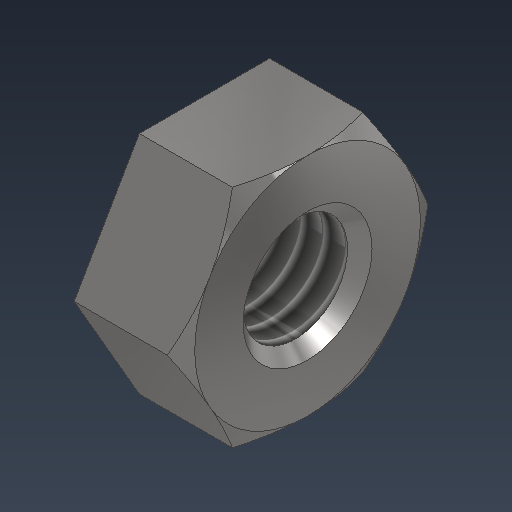
# Autodesk Inventor part: LBNR4
Saved by Autodesk Inventor 2021 (Build 250183000, 183)
## iProperties
Part Number: LBNR4
Material: 鋼、炭素鋼
Catalog Web Link: www.cadenas.de
Description: LBNR, LBNL, SLBNR, SLBNL, KNTR, KNTL, SKNTR-Nuts
Vendor: MISUMI
Document SubType Name: Modeling
Designer: partserver
Manufacturer: MISUMI
Mass: 0.843306 g
Surface Area: 1.72411 cm^2
Volume: 0.107428 cm^3
Density: 7.85 g/cm^3
Appearance: 半つや出し
Category: PARTsolutions
Company: MISUMI
PSOL_IDENT_0: {$CADENAS_DATA\23d-libs\misumi\metric\27_screws_nuts\slbnl.prj},197 {VTYP=3D},{NB=LBNR4},{LINA=LBNR4
PSOL_IDENT_1: },{NN=LBNR, LBNL, SLBNR, SLBNL, KNTR, KNTL, SKNTR},{DATE=09.09.2019 15:27:56},{GEOMDATE=05.11.2010 0
PSOL_IDENT_2: 0:00:00},{VERSION=},{LINEID=30},{WBVAR=TRS,MAT,CS},{WBNUMERIC=}  {NB=LBNR4},{LINA=LBNR4},{KT=DUMMY},
PSOL_IDENT_3: {PN=LBNR4},{TS=LBN},{TRS=R},{MAT=},{ST=Trivalent Chromate},{CS=1},{M1=4},{M=4.0},{P=0.70},{B=7.0},{E
PSOL_IDENT_4: E=8.1},{T=3.2},{T1=0.0},{TFX=3.2},{T1FX=2.4},{CALG='1','JIS Class 1','2','JIS Class 3'},{TRSALG= 'R'
PSOL_IDENT_5: , 'Right-Hand Thread', 'L', 'Left-Hand Thread' },{MATALG= '', 'SWCH Carbon Steel', 'S', '304 Stainle
PSOL_IDENT_6: ss Steel' }
NB: LBNR4
NN: LBNR, LBNL, SLBNR, SLBNL, KNTR, KNTL, SKNTR
NT: Nuts
NBSYN: $PN.
LINA: LBNR4
CATALOG: Misumi
PN: LBNR4
TRS: Right-Hand Thread
MAT: JIS-SWCH Carbon Steel Equivalent
ST: Trivalent Chromate
CS: JIS Class 1
M1: 4
P: 0.7
B: 7
EE: 8.1
T: 3.2
T1: 0
SUPPLIER: MISUMI
ARTICLENO: LBNR4
BOMINFO: LBNR4
CREATOR: CADENAS GmbH
Title: LBNR4
Author: Cadenas PARTsolutions
Comments: Nuts
Autodesk Inventor part; units mm, degrees
sketch "Sketch_1" plane through (0, 0, 0) normal (0, 0, 1) x (1, 0, 0)
  line L0 (1.6, 0) -> (-1.6, 0)
  line L1 (-1.6, 0) -> (-1.6, 3.5)
  line L2 (-1.6, 3.5) -> (-1.2825, 4.05)
  line L3 (-1.2825, 4.05) -> (1.6, 4.05)
  line L4 (1.6, 4.05) -> (1.6, 0)
  line L5 (1.6, 0) -> (-1.6, 0)
  constraints: 12 end point
revolve "Revolution1" add sketch "Sketch_1" angle 360 about axis through (1.6, 0, 0) along (1, 0, 0)
sketch "Sketch_2" plane through (0, 0, 0) normal (0, 0, 1) x (1, 0, 0)
  line L0 (1.6, 0) -> (-1.6, 0)
  line L1 (-1.6, 0) -> (-1.6, 2)
  line L2 (-1.6, 2) -> (-1.221, 1.621)
  line L3 (-1.221, 1.621) -> (1.221, 1.621)
  line L4 (1.221, 1.621) -> (1.6, 2)
  line L5 (1.6, 2) -> (1.6, 0)
  line L6 (1.6, 0) -> (-1.6, 0)
  constraints: 14 end point
revolve "Revolution2" cut sketch "Sketch_2" angle 360 about axis through (1.6, 0, 0) along (1, 0, 0)
thread "Thread1" size "M4x0.7" class "6H" standard "ISO Metric profile" full length
sketch "Sketch_3" plane through (0, 0, 0) normal (1, 0, 0) x (0, 1, 0)
  line L0 (-7, 7) -> (-7, -7)
  line L1 (-7, -7) -> (7, -7)
  line L2 (7, -7) -> (7, 7)
  line L3 (7, 7) -> (-7, 7)
  line L4 (-2.0207, 3.5) -> (-4.0415, 0)
  line L5 (-4.0415, 0) -> (-2.0207, -3.5)
  line L6 (-2.0207, -3.5) -> (2.0207, -3.5)
  line L7 (2.0207, -3.5) -> (4.0415, 0)
  line L8 (4.0415, 0) -> (2.0207, 3.5)
  line L9 (2.0207, 3.5) -> (-2.0207, 3.5)
  constraints: 20 end point
extrude "Extrusion1" cut sketch "Sketch_3" along normal mid plane 3.2
ref_plane "cp_XY" through (1.6, 0, 0) normal (1, 0, 0) x (0, 0, -1)
ref_plane "cp_YZ" through (1.6, 0, 0) normal (0, 0, -1) x (0, 1, 0)
ref_plane "cp_ZX" through (1.6, 0, 0) normal (0, 1, 0) x (1, 0, 0)
ref_plane "nut_to_screw_XY" through (0, 0, 0) normal (1, 0, 0) x (0, 0, -1)
ref_plane "nut_to_screw_YZ" through (0, 0, 0) normal (0, 0, -1) x (0, 1, 0)
ref_plane "nut_to_screw_ZX" through (0, 0, 0) normal (0, 1, 0) x (1, 0, 0)
body "Solid1"
